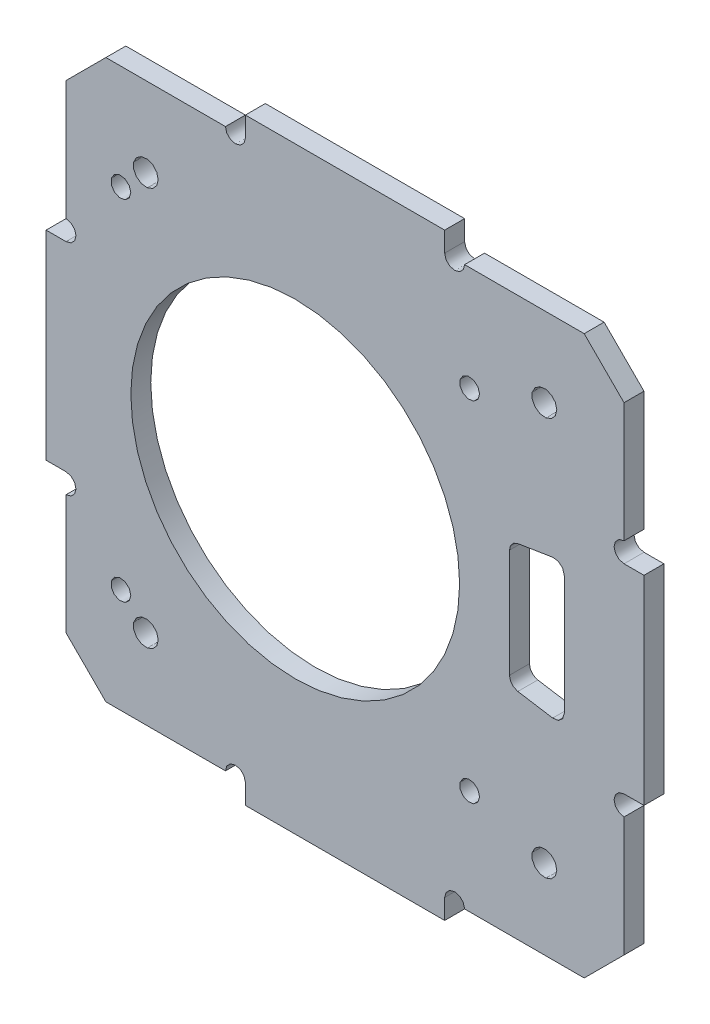
# Autodesk Inventor part: Pieza4
Saved by Autodesk Inventor 2017 (Build 210142000, 142)
## iProperties
Part Number: Pieza4
Material: Genérico
Document SubType Name: Modeling
Designer: Leo
Density: 1 g/cm^3
Appearance: Valor por defecto
Author: Leo
Autodesk Inventor part; units mm, degrees
ref_plane "YZ Plane" through (0, 0, 0) normal (1, 0, 0) x (0, 1, 0)
ref_plane "XZ Plane" through (0, 0, 0) normal (0, 1, 0) x (-1, 0, 0)
ref_plane "XY Plane" through (0, 0, 0) normal (0, 0, 1) x (1, 0, 0)
sketch "Boceto1" plane through (0, 0, 0) normal (0, 0, 1) x (1, 0, 0)
  line L0 (40.5, 8.5) -> (-5.5, 8.5) construction
  line L1 (-5.5, 8.5) -> (-5.5, 32.5) construction
  line L2 (-5.5, 32.5) -> (40.5, 32.5) construction
  line L3 (40.5, 32.5) -> (40.5, 8.5) construction
  line L4 (26.5, -12) -> (26.5, -31) construction
  line L5 (26.5, -31) -> (-0.5, -31) construction
  line L6 (-0.5, -31) -> (-0.5, -12) construction
  line L7 (-0.5, -12) -> (26.5, -12) construction
  circle A0 centre (-40, -40) radius 2.5 projected
  circle A1 centre (-40, 40) radius 2.5 projected
  circle A2 centre (40, 40) radius 2.5 projected
  circle A3 centre (40, -40) radius 2.5 projected
  line L8 (-60, 20) -> (-60, -20) projected
  line L9 (-60, -20) -> (-56, -20) projected
  arc A4 (-56, -24) -> (-56, -20) centre (-56, -22) ccw projected
  line L10 (-56, -24) -> (-56, -48) projected
  line L11 (-56, -48) -> (-48, -56) projected
  line L12 (-48, -56) -> (-24, -56) projected
  arc A5 (-20, -56) -> (-24, -56) centre (-22, -56) ccw projected
  line L13 (-20, -56) -> (-20, -60) projected
  line L14 (-20, -60) -> (20, -60) projected
  line L15 (20, -60) -> (20, -56) projected
  arc A6 (24, -56) -> (20, -56) centre (22, -56) ccw projected
  line L16 (24, -56) -> (48, -56) projected
  line L17 (48, -56) -> (56, -48) projected
  line L18 (56, -48) -> (56, -24) projected
  arc A7 (56, -20) -> (56, -24) centre (56, -22) ccw projected
  line L19 (56, -20) -> (60, -20) projected
  line L20 (60, -20) -> (60, 20) projected
  line L21 (60, 20) -> (56, 20) projected
  arc A8 (56, 24) -> (56, 20) centre (56, 22) ccw projected
  line L22 (56, 24) -> (56, 48) projected
  line L23 (56, 48) -> (48, 56) projected
  line L24 (48, 56) -> (24, 56) projected
  arc A9 (20, 56) -> (24, 56) centre (22, 56) ccw projected
  line L25 (20, 56) -> (20, 60) projected
  line L26 (20, 60) -> (-20, 60) projected
  line L27 (-20, 60) -> (-20, 56) projected
  arc A10 (-24, 56) -> (-20, 56) centre (-22, 56) ccw projected
  line L28 (-24, 56) -> (-48, 56) projected
  line L29 (-48, 56) -> (-56, 48) projected
  line L30 (-56, 48) -> (-56, 24) projected
  arc A11 (-56, 20) -> (-56, 24) centre (-56, 22) ccw projected
  line L31 (-56, 20) -> (-60, 20) projected
  line L32 (25, 35) -> (-45, 35) construction
  line L33 (-45, 35) -> (-45, -35) construction
  line L34 (-45, -35) -> (25, -35) construction
  line L35 (25, -35) -> (25, 35) construction
  circle A12 centre (25, 35) radius 2
  circle A13 centre (25, -35) radius 2
  circle A14 centre (-45, -35) radius 2
  circle A15 centre (-45, 35) radius 2
  circle A16 centre (-10, 0) radius 33
  line L36 (44, 12) -> (44, -12)
  arc A17 (41.6827, -13.9747) -> (44, -12) centre (42, -12) ccw
  line L37 (41.6827, -13.9747) -> (34.6827, -12.85)
  arc A18 (33, -10.8753) -> (34.6827, -12.85) centre (35, -10.8753) ccw
  line L38 (33, -10.8753) -> (33, 10.8753)
  arc A19 (34.6827, 12.85) -> (33, 10.8753) centre (35, 10.8753) ccw
  line L39 (34.6827, 12.85) -> (41.6827, 13.9747)
  arc A20 (44, 12) -> (41.6827, 13.9747) centre (42, 12) ccw
  point P0 (25, 0)
  point P1 (60, 0)
  point P2 (-10, 35)
  point P3 (33, 0)
  point P4 (44, 0)
  dimension "d0" = 70
  dimension "d1" = 4
  dimension "d2" = 66
  dimension "d3" = 2
  dimension "d4" = 11
  dimension "d5" = 28
  dimension "d6" = 25.7
  dimension "d7" = 11
  dimension "d8" = 8
  constraints: 16 end point, 9 centre point, 8 point on circle, 8 tangent, 6 equal radius, 5 midpoint, 4 coincident, 4 horizontal alignment, 3 parallel, 2 perpendicular, 1 horizontal, 1 vertical, 1 vertical alignment
  measures "d0" distance of L32.start L32.end
  measures "d1" diameter of A12
  measures "d2" diameter of A16
  measures "d3" radius of A19
  measures "d4" distance between parallel lines of L36 L38
  measures "d6" distance of L39.start L37.end
  measures "d7" distance between parallel lines of L33 L30
  measures "d8" distance between parallel lines of L38 L35
extrude "Extrusión1" add sketch "Boceto1" along normal blind 4
